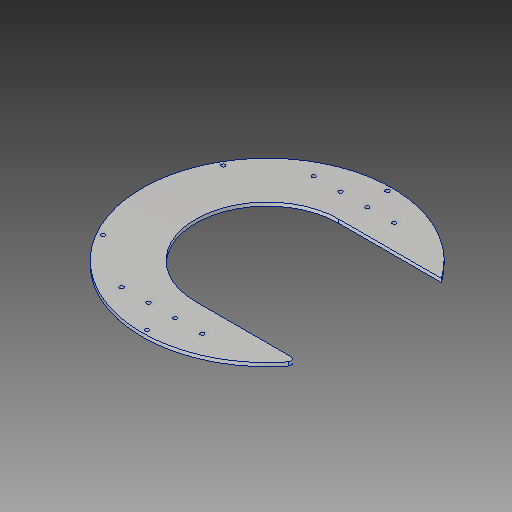
# Autodesk Inventor part: Turret Support
Saved by Autodesk Inventor 2019.4 (Build 234330000, 330)
## iProperties
Created: 2020-01-19
Part Number: Turret Support
Material: Aluminum 6061
Document SubType Name: Modeling
Designer: Mark
Mass: 637.292 g
Surface Area: 1028.47 cm^2
Volume: 236.034 cm^3
Density: 2.7 g/cm^3
Appearance: Aluminum - Flat
Author: Mark
Autodesk Inventor part; units mm, degrees
ref_plane "YZ Plane" through (0, 0, 0) normal (1, 0, 0) x (0, 1, 0)
ref_plane "XZ Plane" through (0, 0, 0) normal (0, 1, 0) x (-1, 0, 0)
ref_plane "XY Plane" through (0, 0, 0) normal (0, 0, 1) x (1, 0, 0)
sketch "Sketch1" plane through (0, 0, 0) normal (0, 1, 0) x (-1, 0, 0)
  circle A0 centre (0, 0) radius 175
  dimension "d0" = 350
  constraints: 1 centre point, 1 coincident
  measures "d0" diameter of A0
extrude "Extrusion1" add sketch "Sketch1" along normal blind 5
sketch "Sketch2" plane through (0, 5, 0) normal (0, 1, 0) x (1, 0, 0)
  ellipse E0 centre (-106.8, 134.3) end of major axis (-106.8, 137.05) minor radius 2.75 construction
  ellipse E1 centre (-69.3001, 134.3) end of major axis (-69.3001, 137.05) minor radius 2.75 projected
  ellipse E2 centre (-31.8001, 134.3) end of major axis (-31.8001, 137.05) minor radius 2.75 projected
  ellipse E3 centre (5.6999, 134.3) end of major axis (5.6999, 137.05) minor radius 2.75 projected
  ellipse E4 centre (43.1998, 134.3) end of major axis (43.1998, 137.05) minor radius 2.75 projected
  constraints: 5 other
extrude "Extrusion2" cut sketch "Sketch2" against normal blind 5
sketch "Sketch3" plane through (0, 5, 0) normal (0, 1, 0) x (1, 0, 0)
  line L0 (-115, 100) -> (0, 100) construction
  line L1 (115, 100) -> (115, -100)
  line L2 (115, -100) -> (0, -100)
  line L3 (-115, -100) -> (-115, 100) construction
  line L4 (-115, 100) -> (115, -100) construction
  line L5 (115, 100) -> (-115, -100) construction
  line L6 (115, 100) -> (235, 100)
  line L7 (235, 100) -> (235, -100)
  line L8 (235, -100) -> (115, -100)
  line L9 (115, -100) -> (115, 100)
  circle A0 centre (0, 0) radius 100
  line L10 (0, 100) -> (115, 100)
  line L11 (0, -100) -> (-115, -100) construction
  circle A1 centre (0, 0) radius 175 projected
  dimension "d17" = 230
  dimension "d18" = 200
  dimension "d19" = 120
  dimension "d20" = 200
  dimension "d34" = 200
  constraints: 24 end point, 7 parallel, 3 horizontal, 3 perpendicular, 2 midpoint, 2 point on circle, 1 centre point, 1 coincident, 1 concentric
  measures "d17" distance of L1.end L3.start
  measures "d18" distance of L1.start L1.end
  measures "d19" distance of L7.end L8.end
  measures "d20" distance of L6.end L7.end
  measures "d34" diameter of A0
extrude "Extrusion3" cut sketch "Sketch3" against normal blind 5 contours L6 A1 L8 L1 | L1 L2 A0 L10 | L6 L7 L8 A1 | A0
fillet "Fillet2" radius 5 1 edges at (143.6141, 2.5, 100)
sketch "Sketch4" plane through (0, 5, 0) normal (0, 1, 0) x (1, 0, 0)
  circle A0 centre (0, 0) radius 168.25 construction
  circle A1 centre (0, 168.25) radius 2.75
  line L0 (0, 0) -> (0, 168.25) construction
  line L1 (0, 0) -> (168.25, 0) construction
  circle A2 centre (-145.7088, 84.125) radius 2.75
  circle A3 centre (-145.7088, -84.125) radius 2.75
  circle A4 centre (0, -168.25) radius 2.75
  circle A5 centre (145.7088, -84.125) radius 2.75
  circle A6 centre (145.7088, 84.125) radius 2.75
  dimension "d25" = 336.5
  dimension "d26" = 5.5
  dimension "d27" = 90
  dimension "d30" = 360
  constraints: 6 centre point, 4 end point, 1 coincident, 1 horizontal, 1 perpendicular, 1 vertical alignment, 15 other
  measures "d26" diameter of A1
  measures "d27" angle of L1 L0
extrude "Extrusion4" cut sketch "Sketch4" against normal blind 10 contours A1 | A2 | A3 | A4 | A6
mirror "Mirror1" about plane through (0, 0, 0) normal (0, 0, 1) of "Extrusion2"
body "Solid1"
